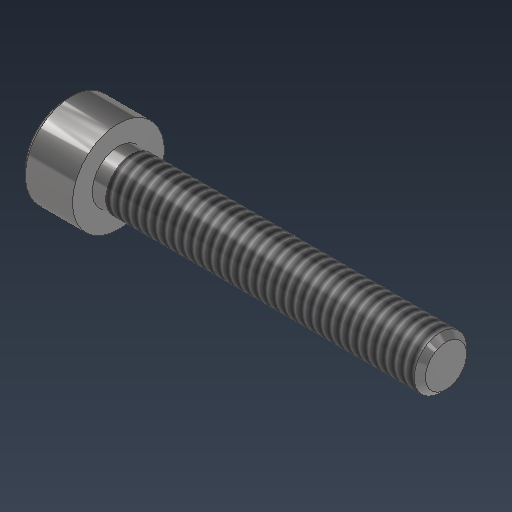
# Autodesk Inventor part: CB4-25
Saved by Autodesk Inventor 2021 (Build 250183000, 183)
## iProperties
Category: PARTsolutions
Company: MISUMI
Created: 2017-11-03
Part Number: CB4-25
Catalog Web Link: www.cadenas.de
Description: CB-Hexagon Socket Head Cap Screws
Vendor: MISUMI
Document SubType Name: Modeling
Designer: psAdmin
Manufacturer: MISUMI
Mass: 3.52303 g
Surface Area: 4.91364 cm^2
Volume: 0.448793 cm^3
Density: 7.85 g/cm^3
Material: 鋼、炭素鋼
Appearance: 半つや出し
PSOL_IDENT_0: {$CADENAS_DATA\23d-libs\misumi\metric\27_screws_nuts\cb_fa.prj},151 {VTYP=3D},{NB=CB4-25},{LINA=CB4-
PSOL_IDENT_1: 25},{NN=CB},{DATE=24.04.2017 09:49:34},{GEOMDATE=17.02.2014 00:00:00},{VERSION=},{LINEID=50},{LINESU
PSOL_IDENT_2: BID=-1},{WBVAR=L}  {NB=CB4-25},{LINA=CB4-25},{KT=DUMMY},{PN=CB4-25},{MAT=4137 Steel},{HARD=38~43HRC}
PSOL_IDENT_3: ,{ST=Black Oxide},{M=4},{L=25},{LL=Full Thread},{L1=20},{TYPE=CB},{M1=4.000},{L0=5,6,8,10,12,14,15,1
PSOL_IDENT_4: 6,18,20,22,25,30,35,40,45,50,55,60},{NDM=4},{KDM=3.139931},{MP=4x0.7},{P=0.7},{A=7.0},{E=4.0},{B=3.0
PSOL_IDENT_5: },{V=0.4}
NN: CB
NT: Hexagon Socket Head Cap Screws
NB: CB4-25
NBSYN: $PN.
LINA: CB4-25
PN: CB4-25
MAT: 4137 Steel
HARD: 38~43HRC
ST: Black Oxide
M: 4
L: 25
LL: Full Thread
MP: 4x0.7
A: 7.0
E: 4.0
B: 3.0
SUPPLIER: MISUMI
ARTICLENO: CB4-25
BOMINFO: CB4-25
CREATOR: CADENAS GmbH
購入先: ミスミ
在庫数: 0.0
Title: CB4-25
Author: Cadenas PARTsolutions
Comments: Hexagon Socket Head Cap Screws
Autodesk Inventor part; units mm, degrees
sketch "Sketch_1" plane through (0, 0, 0) normal (0, 0, 1) x (1, 0, 0)
  line L0 (25, 0) -> (-4, 0)
  line L1 (-4, 0) -> (-4, 3.1)
  line L2 (-4, 3.1) -> (-3.6, 3.5)
  line L3 (-3.6, 3.5) -> (0, 3.5)
  line L4 (0, 3.5) -> (0, 2)
  line L5 (0, 2) -> (24.5705, 2)
  line L6 (24.5705, 2) -> (25, 1.5705)
  line L7 (25, 1.5705) -> (25, 0)
  line L8 (25, 0) -> (-4, 0)
  constraints: 18 end point
revolve "Revolution1" add sketch "Sketch_1" angle 360 about axis through (25, 0, 0) along (1, 0, 0)
thread "Thread1" size "M4x0.7" class "6g" standard "ISO Metric profile" length 24 offset 1
sketch "Sketch_4_ALT_Drilling_1" plane through (0, 0, 0) normal (0, 0, 1) x (1, 0, 0)
  line L0 (-1.5981, 0) -> (-4, 0)
  line L1 (-4, 0) -> (-4, 1.5)
  line L2 (-4, 1.5) -> (-2, 1.5)
  line L3 (-2, 1.5) -> (-1.5981, 0)
  line L4 (-1.5981, 0) -> (-4, 0)
  constraints: 10 end point
revolve "Revolution2" cut sketch "Sketch_4_ALT_Drilling_1" angle 360 about axis through (-1.5981, 0, 0) along (1, 0, 0)
sketch "Sketch_3" plane through (-4, 0, 0) normal (1, 0, 0) x (0, 0, -1)
  line L0 (-1.5, -0.866) -> (0, -1.7321)
  line L1 (0, -1.7321) -> (1.5, -0.866)
  line L2 (1.5, -0.866) -> (1.5, 0.866)
  line L3 (1.5, 0.866) -> (0, 1.7321)
  line L4 (0, 1.7321) -> (-1.5, 0.866)
  line L5 (-1.5, 0.866) -> (-1.5, -0.866)
  constraints: 12 end point
extrude "Extrusion1" cut sketch "Sketch_3" along normal blind 2
ref_plane "bolt_to_nut_XY" through (25, 0, 0) normal (1, 0, 0) x (0, 0, -1)
ref_plane "bolt_to_nut_YZ" through (25, 0, 0) normal (0, 0, -1) x (0, 1, 0)
ref_plane "bolt_to_nut_ZX" through (25, 0, 0) normal (0, 1, 0) x (1, 0, 0)
ref_plane "screw1_XY" through (0, 0, 0) normal (1, 0, 0) x (0, 0, -1)
ref_plane "screw1_YZ" through (0, 0, 0) normal (0, 0, -1) x (0, 1, 0)
ref_plane "screw1_ZX" through (0, 0, 0) normal (0, 1, 0) x (1, 0, 0)
body "Solid1"
